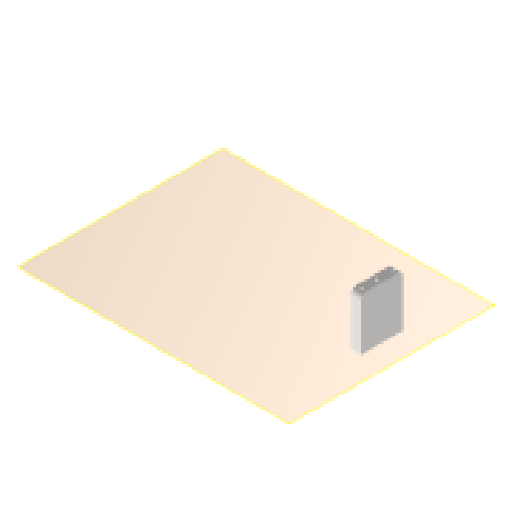
# Autodesk Inventor part: 60_Planktoscope_Illuminationsource
Saved by Autodesk Inventor 2024.1 (Build 281209000, 209)
## iProperties
Created: 2024-07-24
Part Number: 60_Planktoscope_Illuminationsource
Material: Generisch
Document SubType Name: Modeling
Designer: diederichbenedict
Density: 1 g/cm^3
Appearance: Vorgabe
Author: diederichbenedict
Autodesk Inventor part; units mm, degrees
ref_plane "YZ Plane" through (0, 0, 0) normal (1, 0, 0) x (0, 1, 0)
ref_plane "XZ Plane" through (0, 0, 0) normal (0, 1, 0) x (-1, 0, 0)
ref_plane "XY Plane" through (0, 0, 0) normal (0, 0, 1) x (1, 0, 0)
ref_plane "Arbeitsebene1" through (0, 0, 0) normal (0, 0, 1) x (1, 0, 0)
sketch "Skizze1" plane through (0, 0, 0) normal (0, 0, 1) x (1, 0, 0)
  line L0 (-118.5, -74.5) -> (-118.5, 74.5) projected
  arc A0 (-118.5, -74.5) -> (-103.5, -89.5) centre (-103.5, -74.5) ccw projected
  line L1 (56.1, -89.5) -> (-103.5, -89.5) projected
  line L2 (56.1, -83) -> (56.1, -89.5) projected
  arc A1 (71.1, -68) -> (56.1, -83) centre (71.1, -83) ccw projected
  line L3 (80.5, -68) -> (71.1, -68) projected
  arc A2 (95.5, -83) -> (80.5, -68) centre (80.5, -83) ccw projected
  line L4 (95.5, -89.5) -> (95.5, -83) projected
  line L5 (103.5, -89.5) -> (95.5, -89.5) projected
  arc A3 (103.5, -89.5) -> (118.5, -74.5) centre (103.5, -74.5) ccw projected
  line L6 (118.5, 74.5) -> (118.5, -74.5) projected
  arc A4 (118.5, 74.5) -> (103.5, 89.5) centre (103.5, 74.5) ccw projected
  line L7 (-103.5, 89.5) -> (103.5, 89.5) projected
  arc A5 (-103.5, 89.5) -> (-118.5, 74.5) centre (-103.5, 74.5) ccw projected
  circle A6 centre (-58.5, 18.7) radius 1.4 projected
  circle A7 centre (-58.5, 36.552) radius 1.4 projected
  circle A8 centre (57.5, 20.252) radius 1.4 projected
  circle A9 centre (57.5, 35) radius 1.4 projected
  circle A10 centre (-58.5, 8.7) radius 1.4 projected
  circle A11 centre (-58.5, -9.152) radius 1.4 projected
  circle A12 centre (57.5, 7.148) radius 1.4 projected
  circle A13 centre (57.5, -7.6) radius 1.4 projected
  circle A14 centre (103.5, 74.5) radius 1.4 projected
  circle A15 centre (103.5, -74.5) radius 1.4 projected
  circle A16 centre (-103.5, -74.5) radius 1.4 projected
  circle A17 centre (-103.5, 74.5) radius 1.4 projected
  line L8 (20.9567, 0.5738) -> (-20.9567, 0.5738) projected
  line L9 (-20.9567, 0.5738) -> (-20.9567, 30.6837) projected
  line L10 (-20.9567, 30.6837) -> (20.9567, 30.6837) projected
  line L11 (20.9567, 30.6837) -> (20.9567, 0.5738) projected
  circle A18 centre (73.1917, -22.4328) radius 1.4 projected
  circle A19 centre (43.1917, -22.4328) radius 1.4 projected
  circle A20 centre (13.1917, -22.4328) radius 1.4 projected
  circle A21 centre (-16.8083, -22.4328) radius 1.4 projected
  circle A22 centre (-46.8083, -22.4328) radius 1.4 projected
  circle A23 centre (-102.338, -1.3) radius 1.4 projected
  circle A24 centre (-102.338, 13.7) radius 1.4 projected
  circle A25 centre (-102.338, 28.7) radius 1.4 projected
  circle A26 centre (102.338, 28.7) radius 1.4 projected
  circle A27 centre (-73.1917, -22.4328) radius 1.4 projected
  circle A28 centre (-43.1917, -22.4328) radius 1.4 projected
  circle A29 centre (-13.1917, -22.4328) radius 1.4 projected
  circle A30 centre (16.8083, -22.4328) radius 1.4 projected
  circle A31 centre (46.8083, -22.4328) radius 1.4 projected
  circle A32 centre (102.338, -1.3) radius 1.4 projected
  circle A33 centre (102.338, 13.7) radius 1.4 projected
  line L12 (97.338, -6.3) -> (107.338, -6.3)
  line L13 (107.338, -6.3) -> (107.338, 33.7)
  line L14 (107.338, 33.7) -> (97.338, 33.7)
  line L15 (97.338, 33.7) -> (97.338, -6.3)
  line L16 (97.338, -6.3) -> (107.338, 33.7) construction
  line L17 (107.338, -6.3) -> (97.338, 33.7) construction
  point P0 (0, 0)
  dimension "d0" = 10
  dimension "d1" = 40
  constraints: 12 end point, 2 midpoint, 2 parallel, 1 horizontal, 1 perpendicular
  measures "d0" distance of L14.end L13.end
  measures "d1" distance of L13.end L12.end
extrude "Extrusion1" add sketch "Skizze1" along normal blind 50 contours L15 L14 L13 L12
fillet "Rundung1" radius 5 2 edges at (102.338, -6.3, 50) (102.338, 33.7, 50)
